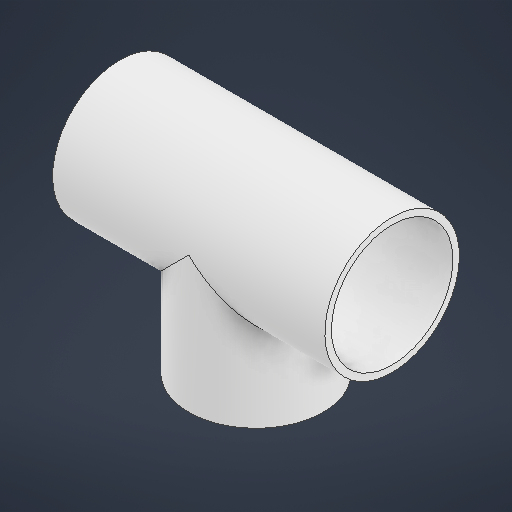
# Autodesk Inventor part: Connector
Saved by Autodesk Inventor 2027 (Build 310192000, 192)
## iProperties
Created: 2026-04-30
Part Number: Connector
Material: PVC-Piping
Document SubType Name: Modeling
Designer: bhoga
Density: 1.4 g/cm^3
Appearance: Smooth - White
Author: bhoga
Autodesk Inventor part; units mm, degrees
ref_plane "YZ Plane" through (0, 0, 0) normal (1, 0, 0) x (0, 1, 0)
ref_plane "XY Plane" through (0, 0, 0) normal (0, 0, 1) x (1, 0, 0)
sketch "Sketch1" plane through (0, 0, 0) normal (1, 0, 0) x (0, 1, 0)
  circle A0 centre (0, 0) radius 11.15
  circle A1 centre (0, 0) radius 12.3475
  dimension "d0" = 22.3
  dimension "d1" = 24.695
  constraints: 2 centre point, 2 coincident
  measures "d0" diameter of A0
  measures "d1" diameter of A1
extrude "Extrusion1" add sketch "Sketch1" along normal blind 50
ref_plane "Work Plane2" through (0, -25, 0) normal (0, 1, 0) x (-1, 0, 0)
sketch "Sketch2" plane through (0, -25, 0) normal (0, 1, 0) x (-1, 0, 0)
  line L0 (0, 0) -> (-50, 0)
  line L1 (-50, 12.3475) -> (-50, -12.3475) projected
  circle A0 centre (-25, 0) radius 12.3475
  circle A1 centre (-25, 0) radius 11.15
  dimension "d6" = 50
  dimension "d7" = 22.3
  constraints: 2 centre point, 2 end point, 2 midpoint, 1 coincident
  measures "d6" distance of L0.start L0.end
  measures "d7" diameter of A1
extrude "Extrusion2" add sketch "Sketch2" along normal blind 25 contours A0 L0 A1 | L0 A1 A0
sketch "Sketch3" plane through (0, 0, 0) normal (-1, 0, 0) x (0, 0, 1)
  line L0 (11.15, 0) -> (-11.15, 0) projected
  circle A0 centre (0, 0) radius 11.15
  constraints: 1 coincident, 1 horizontal alignment, 2 other
extrude "Extrusion3" cut sketch "Sketch3" against normal blind 78.975
sketch "Sketch4" plane through (25, -25, 0) normal (0, -1, 0) x (1, 0, 0)
  circle A0 centre (0, 0) radius 11.15
  point P0 (-25, 0)
  constraints: 1 centre point
extrude "Extrusion4" cut sketch "Sketch4" against normal blind 25
body "Solid1"
